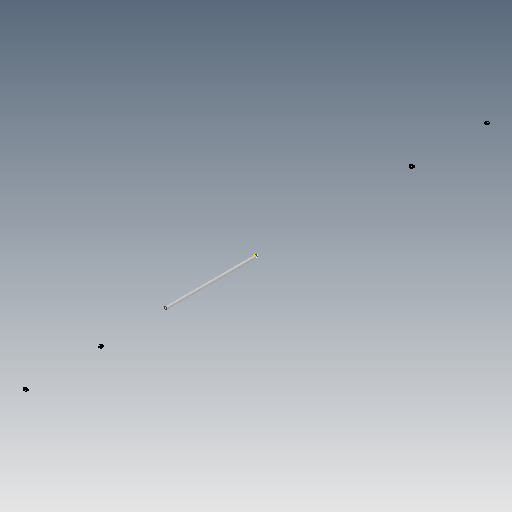
# Autodesk Inventor part: 365 Mono
Saved by Autodesk Inventor 2017 (Build 210142000, 142)
## iProperties
Created: 2019-06-06
Part Number: 365 Mono
Material: Generic
Document SubType Name: Modeling
Designer: Admin
Density: 1 g/cm^3
Appearance: Default
Mass: 28.667 g
Surface Area: 116.239 cm^2
Volume: 28.667 cm^3
Author: Admin
Autodesk Inventor part; units mm, degrees
ref_plane "YZ Plane" through (0, 0, 0) normal (1, 0, 0) x (0, 1, 0)
ref_plane "XZ Plane" through (0, 0, 0) normal (0, 1, 0) x (-1, 0, 0)
ref_plane "XY Plane" through (0, 0, 0) normal (0, 0, 1) x (1, 0, 0)
sketch "Sketch1" plane through (0, 0, 0) normal (0, 0, 1) x (1, 0, 0)
  circle A0 centre (0, 0) radius 5
  dimension "d0" = 10
  constraints: 1 centre point, 1 coincident
  measures "d0" diameter of A0
extrude "Extrusion1" add sketch "Sketch1" along normal blind 365
sketch "Sketch2" plane through (0, 0, 0) normal (0, 1, 0) x (-1, 0, 0)
  line L0 (-4.3053, -632.2581) -> (4.3053, -632.2581)
  line L1 (4.3053, -632.2581) -> (4.3053, -621.4108)
  line L2 (4.3053, -621.4108) -> (-4.3053, -621.4108)
  line L3 (-4.3053, -621.4108) -> (-4.3053, -632.2581)
  line L4 (-4.3053, -632.2581) -> (4.3053, -621.4108) construction
  line L5 (4.3053, -632.2581) -> (-4.3053, -621.4108) construction
  line L6 (-4.3053, -933.664) -> (4.3053, -933.664)
  line L7 (4.3053, -933.664) -> (4.3053, -925.5918)
  line L8 (4.3053, -925.5918) -> (-4.3053, -925.5918)
  line L9 (-4.3053, -925.5918) -> (-4.3053, -933.664)
  line L10 (-4.3053, -933.664) -> (4.3053, -925.5918) construction
  line L11 (4.3053, -933.664) -> (-4.3053, -925.5918) construction
  line L12 (-4.3053, 632.2581) -> (4.3053, 632.2581)
  line L13 (4.3053, 632.2581) -> (4.3053, 621.4108)
  line L14 (4.3053, 621.4108) -> (-4.3053, 621.4108)
  line L15 (-4.3053, 621.4108) -> (-4.3053, 632.2581)
  line L16 (-4.3053, 632.2581) -> (4.3053, 621.4108) construction
  line L17 (4.3053, 632.2581) -> (-4.3053, 621.4108) construction
  line L18 (-4.3053, 933.664) -> (4.3053, 933.664)
  line L19 (4.3053, 933.664) -> (4.3053, 925.5918)
  line L20 (4.3053, 925.5918) -> (-4.3053, 925.5918)
  line L21 (-4.3053, 925.5918) -> (-4.3053, 933.664)
  line L22 (-4.3053, 933.664) -> (4.3053, 925.5918) construction
  line L23 (4.3053, 933.664) -> (-4.3053, 925.5918) construction
  point P0 (0, 0)
  point P1 (0, -626.8344)
  point P2 (0, -929.6279)
  point P3 (0, 626.8344)
  point P4 (0, 929.6279)
  constraints: 48 end point, 8 midpoint, 4 parallel, 2 horizontal, 2 perpendicular, 2 point on line
body "Solid1"
